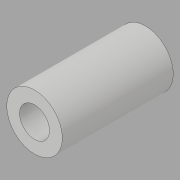
# Autodesk Inventor part: Top Spacer
Saved by Autodesk Inventor 2017 (Build 210142000, 142)
## iProperties
Created: 2022-08-18
Part Number: Top Spacer
Material: Generic
Document SubType Name: Modeling
Designer: JTS
Density: 1 g/cm^3
Appearance: Default
Author: JTS
Autodesk Inventor part; units mm, degrees
ref_plane "YZ Plane" through (0, 0, 0) normal (1, 0, 0) x (0, 1, 0)
ref_plane "XZ Plane" through (0, 0, 0) normal (0, 1, 0) x (-1, 0, 0)
ref_plane "XY Plane" through (0, 0, 0) normal (0, 0, 1) x (1, 0, 0)
sketch "Sketch1" plane through (0, 0, 0) normal (0, 0, 1) x (1, 0, 0)
  circle A0 centre (0, 0) radius 3.429
  circle A1 centre (0, 0) radius 6.35
  dimension "d0" = 12.7
  dimension "d1" = 6.858
  constraints: 2 centre point, 2 coincident
  measures "d0" diameter of A1
  measures "d1" diameter of A0
extrude "Extrusion1" add sketch "Sketch1" along normal blind 25.4
body "Solid1"
